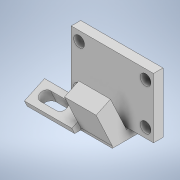
# Autodesk Inventor part: cam mount prototype
Saved by Autodesk Inventor 2022.6 (Build 266554000, 554)
## iProperties
Created: 2024-11-21
Part Number: cam mount prototype
Material: Generic
Document SubType Name: Modeling
Designer: Admin
Density: 1 g/cm^3
Appearance: Default
Author: Admin
Autodesk Inventor part; units mm, degrees
ref_plane "YZ Plane" through (0, 0, 0) normal (1, 0, 0) x (0, 1, 0)
ref_plane "XZ Plane" through (0, 0, 0) normal (0, 1, 0) x (-1, 0, 0)
ref_plane "XY Plane" through (0, 0, 0) normal (0, 0, 1) x (1, 0, 0)
sketch "Sketch2" plane through (0, 0, 0) normal (0, 0, 1) x (1, 0, 0)
  line L0 (-13, -9.5) -> (13, -9.5)
  line L1 (13, -9.5) -> (13, 9.5)
  line L2 (13, 9.5) -> (-13, 9.5)
  line L3 (-13, 9.5) -> (-13, -9.5)
  line L4 (-13, -9.5) -> (13, 9.5) construction
  line L5 (13, -9.5) -> (-13, 9.5) construction
  point P0 (0, 0)
  dimension "d2" = 26
  dimension "d3" = 19
  constraints: 12 end point, 2 midpoint, 2 parallel, 1 horizontal, 1 perpendicular
  measures "d2" distance of L0.start L0.end
  measures "d3" distance of L1.end L0.end
extrude "Extrusion1" add sketch "Sketch2" along normal blind 3
sketch "Sketch1" plane through (0, 0, 0) normal (0, 0, 1) x (1, 0, 0)
  line L0 (-10.5, -6.5) -> (10.5, -6.5) construction
  line L1 (10.5, -6.5) -> (10.5, 6.5) construction
  line L2 (10.5, 6.5) -> (-10.5, 6.5) construction
  line L3 (-10.5, 6.5) -> (-10.5, -6.5) construction
  line L4 (-10.5, -6.5) -> (10.5, 6.5) construction
  line L5 (10.5, -6.5) -> (-10.5, 6.5) construction
  point P0 (0, 0)
  dimension "d0" = 21
  dimension "d1" = 13
  constraints: 12 end point, 2 midpoint, 2 parallel, 1 horizontal, 1 perpendicular
  measures "d0" distance of L1.end L2.end
  measures "d1" distance of L0.end L1.end
hole "Hole1" at (10.5, 6.5, 0) at (-10.5, 6.5, 0) at (10.5, -6.5, 0) at (-10.5, -6.5, 0) direction (0, 0, 1) diameter 3.4 end through all
sketch "Sketch3" plane through (0, 0, 0) normal (1, 0, 0) x (0, 1, 0)
  line L0 (-9.5, 0) -> (9.5, 0) projected
  line L1 (9.5, 0) -> (9.5, 3) projected
  line L2 (-9.5, 3) -> (9.5, 3) projected
  line L3 (-9.5, 0) -> (-9.5, 3) projected
  line L4 (-9.5, 0) -> (9.5, 0) projected
  line L5 (-9.5, 0) -> (-9.5, 8)
  line L6 (-9.5, 8) -> (-12.5, 8)
  line L7 (-12.5, 8) -> (-12.5, 0)
  line L8 (-12.5, 0) -> (-9.5, 0)
  line L9 (-9.5, 8) -> (-0.4369, 12.2262)
  line L10 (-0.4369, 12.2262) -> (1.2536, 8.601)
  line L11 (1.2536, 8.601) -> (-7.8095, 4.3748)
  line L12 (-7.8095, 4.3748) -> (-9.5, 8)
  line L13 (-9.5, 8) -> (0.5, 8) construction
  line L14 (-7.8095, 4.3748) -> (-9.5, 3.5865)
  line L15 (-0.4369, 12.2262) -> (-9.5, 8)
  line L16 (-9.5, 8) -> (-9.9226, 8.9063)
  line L17 (-9.9226, 8.9063) -> (-0.8595, 13.1325)
  line L18 (-0.8595, 13.1325) -> (-0.4369, 12.2262)
  line L19 (-9.9226, 8.9063) -> (-11.8662, 8)
  point P0 (0, 0)
  point P1 (-11, 8)
  dimension "d13" = 3
  dimension "d14" = 8
  dimension "d15" = 25
  dimension "d16" = 4
  dimension "d17" = 10
  dimension "d20" = 1
  dimension "d21" = 2.1445
  constraints: 30 end point, 8 equal length, 4 perpendicular, 3 point on line, 1 horizontal, 1 midpoint
  measures "d13" distance between parallel lines of L7 L5
  measures "d14" distance from line of L8 point (-11, 8)
  measures "d15" angle of L13 L9
  measures "d16" distance of L9.end L10.end
  measures "d17" distance of L5.end L9.end
  measures "d20" distance of L5.end L16.end
  measures "d21" distance of L16.end L19.end
extrude "Extrusion2" add sketch "Sketch3" along normal mid plane 10 contours L8 L7 L6 L5 L3 | L5 L12 L14 | L16 L17 L18 L9 | L9 L10 L11 L12 | L6 L19 L16
sketch "Sketch4" plane through (-5, 0, 0) normal (-1, 0, 0) x (0, 0, 1)
  line L0 (8.601, 1.2536) -> (3.5865, -9.5) projected
  line L1 (13.1325, -0.8595) -> (8, -11.8662) projected
  line L2 (4.4408, -7.668) -> (2.1876, -12.5)
  line L3 (0, -12.5) -> (8, -12.5) projected
  line L4 (9.5697, -8.5) -> (7.7045, -12.5)
  line L5 (7.7045, -12.5) -> (2.1876, -12.5)
  line L6 (4.4408, -7.668) -> (8.9723, -9.7811)
  line L7 (13.1325, -0.8595) -> (8.601, 1.2536) projected
  line L8 (8.9723, -9.7811) -> (10.7849, -10.6263)
  line L9 (10.7849, -10.6263) -> (9.9112, -12.5)
  line L10 (9.9112, -12.5) -> (7.7045, -12.5)
  line L11 (8, -11.8662) -> (8, -12.5) projected
  point P0 (0, 0)
  point P1 (8, -11.8662)
  point P2 (8, -11.8662)
  dimension "d25" = 3
  dimension "d33" = 2
  constraints: 14 end point, 4 collinear, 4 point on line, 2 parallel, 1 perpendicular
  measures "d25" distance from line of L4.end L6
  measures "d33" distance from line of L4 L9.end
extrude "Extrusion3" add sketch "Sketch4" along normal blind 15 contours L6 L1 L4 L3 L2 L0 | L8 L9 L10 L11 L1 | L11 L3 L4
sketch "Sketch6" plane through (-20, -7.668, 4.4408) normal (0, 0.9063, 0.4226) x (1, 0, 0)
  line L0 (3.5, -3.5) -> (8.5, -3.5) construction
  line L1 (3.5, -5.2) -> (8.5, -5.2)
  line L2 (8.5, -1.8) -> (3.5, -1.8)
  arc A0 (3.5, -1.8) -> (3.5, -5.2) centre (3.5, -3.5) ccw
  arc A1 (8.5, -5.2) -> (8.5, -1.8) centre (8.5, -3.5) ccw
  line L3 (0, -7) -> (0, 0) projected
  point P0 (20, 7.2653)
  point P1 (6, -3.5)
  point P2 (0, -3.5)
  dimension "d34" = 5
  dimension "d35" = 3.4
  dimension "d36" = 6
  constraints: 8 end point, 4 point on circle, 4 tangent, 2 centre point, 2 midpoint, 1 horizontal, 1 horizontal alignment, 1 parallel
  measures "d34" distance of L0.start L0.end
  measures "d35" diameter of A1
  measures "d36" distance from line of L3 point (6, -3.5)
extrude "Extrusion5" cut sketch "Sketch6" against normal through all
body "Solid1"
